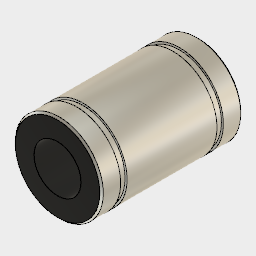
bondtech_x_carriage_mk2s_mk2.5 (Autodesk Fusion 360 archive; units mm, degrees)
design "lm8uu"
Autodesk Fusion 360 part; units mm, degrees
sketch "Sketch1" plane through (0, 0, 0) normal (0, 1, 0) x (1, 0, 0)
  circle A0 centre (0, 0) radius 4
  circle A1 centre (0, 0) radius 7.5
  circle A2 centre (0, 0) radius 7.15
  dimension "d1" = 8
  dimension "d2" = 15
  dimension "d6" = 0.35
  measures "d1" diameter of A0
  measures "d2" diameter of A1
  measures "d6" distance of A1 A2
extrude "Extrude1" add sketch "Sketch1" along normal blind 24 contours A1 | A2
extrude "Extrude2" cut sketch "Sketch1" along normal blind 1.1 from surface at 3.25 contours A1
extrude "Extrude3" cut sketch "Sketch1" against normal blind 1.1 from surface at 20.75 contours A1
chamfer "Chamfer1" distance 0.3 angle 45 2 edges at (-6.9925, 0, 2.7121) (-6.9925, 24, 2.7121)
